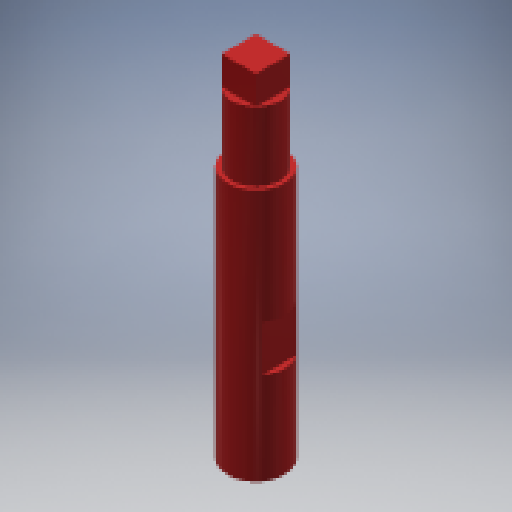
# Autodesk Inventor part: 24_0497_009
Saved by Autodesk Inventor 2024.3 (Build 283343000, 343)
## iProperties
Created: 2024-06-11
Part Number: 24_0497_009
Material: Allgemein
Document SubType Name: Modeling
Designer: Vogel
Density: 1 g/cm^3
Appearance: Hellrot
Author: Vogel
Autodesk Inventor part; units mm, degrees
ref_plane "YZ Plane" through (0, 0, 0) normal (1, 0, 0) x (0, 1, 0)
ref_plane "XZ Plane" through (0, 0, 0) normal (0, 1, 0) x (-1, 0, 0)
ref_plane "XY Plane" through (0, 0, 0) normal (0, 0, 1) x (1, 0, 0)
sketch "Skizze1" plane through (0, 0, 0) normal (0, 0, 1) x (1, 0, 0)
  line L0 (-7, 0) -> (7, 0) projected
  line L1 (0, -7) -> (0, 7) projected
  circle A0 centre (0, 0) radius 5
  dimension "d0" = 10
  constraints: 1 centre point, 1 coincident
  measures "d0" diameter of A0
extrude "Extrusion1" add sketch "Skizze1" along normal blind 44
sketch "Skizze2" plane through (0, 0, 44) normal (0, 0, 1) x (1, 0, 0)
  circle A0 centre (0, 0) radius 5 projected
  circle A1 centre (0, 0) radius 4.25
  dimension "d3" = 8.5
  constraints: 1 centre point, 1 coincident
  measures "d3" diameter of A1
extrude "Extrusion2" add sketch "Skizze2" along normal blind 11 contours A1
sketch "Skizze3" plane through (0, 0, 0) normal (0, 0, -1) x (-1, 0, 0)
  circle A0 centre (0, 0) radius 5 projected
  constraints: 1 coincident
hole "Bohrung1" at (0, 0, 0) direction (0, 0, 1) diameter 4.134 depth 14.2 tip angle 118 thread size "M5x0.8" class "6H" standard "ISO Metric profile"
sketch "Skizze4" plane through (0, 0, 55) normal (0, 0, 1) x (1, 0, 0)
  line L0 (3, -3) -> (-3, -3)
  line L1 (-3, -3) -> (-3, 3)
  line L2 (-3, 3) -> (3, 3)
  line L3 (3, 3) -> (3, -3)
  circle A0 centre (0, 0) radius 4.25 projected
  line L4 (3, -3) -> (-3, 3) construction
  line L5 (-3, -3) -> (3, 3) construction
  dimension "d13" = 6
  dimension "d14" = 6
  constraints: 12 end point, 2 midpoint, 2 parallel, 1 horizontal, 1 perpendicular
  measures "d13" distance of L0.end L1.end
  measures "d14" distance of L1.end L2.end
extrude "Extrusion3" add sketch "Skizze4" along normal blind 5 contours L0 L1 L2 L3
sketch "Skizze5" plane through (0, 0, 0) normal (0, 1, 0) x (-1, 0, 0)
  line L0 (0, -12.3) -> (0, 73.8) projected
  line L1 (7, 0) -> (-7, 0) projected
  line L2 (8.228, 20) -> (-9.772, 20)
  line L3 (5, 44) -> (-5, 44) projected
  line L4 (5, 0) -> (-5, 0) projected
  line L5 (5, 0) -> (5, 44) projected
  line L6 (-5, 0) -> (-5, 44) projected
  line L7 (4, 16) -> (5, 16)
  line L8 (5, 16) -> (5, 24)
  line L9 (5, 24) -> (4, 24)
  line L10 (4, 24) -> (4, 16)
  line L11 (4, 16) -> (5, 24) construction
  line L12 (5, 16) -> (4, 24) construction
  line L13 (-4, 16) -> (-5, 16)
  line L14 (-5, 16) -> (-5, 24)
  line L15 (-5, 24) -> (-4, 24)
  line L16 (-4, 24) -> (-4, 16)
  line L17 (-4, 16) -> (-5, 24) construction
  line L18 (-5, 16) -> (-4, 24) construction
  point P0 (0, 0)
  point P1 (4.5, 20)
  point P2 (-4.5, 20)
  dimension "d17" = 8
  dimension "d18" = 8
  dimension "d19" = 20
  constraints: 26 end point, 5 parallel, 4 midpoint, 3 horizontal, 3 point on line, 2 perpendicular, 1 collinear, 1 other
  measures "d17" distance between parallel lines of L16 L10
  measures "d18" distance of L9.end L7.start
  measures "d19" distance between parallel lines of L1 L2
extrude "Extrusion4" cut sketch "Skizze5" along normal mid plane 44 contours L10 L9 L5 L2 | L2 L5 L7 L10 | L16 L13 L6 L2 | L2 L6 L15 L16
equation "\"d13\" = d14"
